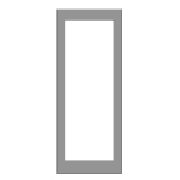
# Autodesk Inventor part: 50x40x3
Saved by Autodesk Inventor 2021 (Build 250183000, 183)
## iProperties
IsCustomPart: 1
Created: 2021-01-06
Part Number: 50x40x3
Material: Aluminum 6061
Document SubType Name: Modeling
Standard: Unnamed
Designer: lucky
Language: en-US
Size Designation: 50 x40 x3
Categories: <MemberInstance><Categories><Category DisplayName="Structural Shapes" InternalName="089c4875-fa83-4c05-b084-43b9cc11f5ed" Mnemonic="GRDR"><CategoryParameter DisplayName="Mass per Length Unit" InternalName="0bb95a10-148f-4027-a459-38d7b056702a" Mnemonic="shpmass"/><CategoryParameter DisplayName="Section Area" InternalName="1ff91680-64b0-4202-b9a3-7fd3f94bba3b" Mnemonic="secarea"/><CategoryParameter DisplayName="Radius of Gyration (x)" InternalName="25778675-03e9-40c1-b6a8-4a9ed693320d" Mnemonic="gyrradx"/><CategoryParameter DisplayName="Torsional Rigidity Modulus" InternalName="26c1ec35-5026-4c63-ad0a-751cf684a536" Mnemonic="torrigmod"/><CategoryParameter DisplayName="Distance of the Center of Gravity X-X" InternalName="26c9bdb8-9c79-4b4f-a92e-8e197583c9c4" Mnemonic="grcendistX"/><CategoryParameter DisplayName="Legacy Member ID" InternalName="340afe4f-75d7-48d3-ab7d-943f3c3da468" Mnemonic="LegacyMemberID"/><CategoryParameter DisplayName="Base Length" InternalName="42e34263-8f20-4d0e-ad48-bf1385b87c24" Mnemonic="shplen"/><CategoryParameter DisplayName="Moment of Inertia (y)" InternalName="4b9f58ea-bced-460e-81ea-3d29ca5a49e3" Mnemonic="inermomy"/><CategoryParameter DisplayName="Moment of Inertia (x)" InternalName="4cd780bc-73d7-43ac-917a-579e5cbd684d" Mnemonic="inermomx"/><CategoryParameter DisplayName="Custom Base Point" InternalName="4f1d1b73-316d-484b-a3df-9cbabb16eb77" Mnemonic="shpBasePoint"/><CategoryParameter DisplayName="Shape Height" InternalName="50274e7d-5ac0-4796-92cb-c59e54983c67" Mnemonic="shpheig"/><CategoryParameter DisplayName="Section Module (y)" InternalName="59eaa5e9-d227-48dc-b6c1-6920f96e0f95" Mnemonic="secmody"/><CategoryParameter DisplayName="Section Designation" InternalName="5a64d034-428d-49c8-ba32-7619764de20f" Mnemonic="shpdes"/><CategoryParameter DisplayName="Section Module (x)" InternalName="72cfad18-cf51-4ed4-aaa7-c6b224f8419f" Mnemonic="secmodx"/><CategoryParameter DisplayName="Torsional Section Modulus" InternalName="7c55a8dc-8844-49f9-a867-cc677b30ec9a" Mnemonic="torsecmod"/><CategoryParameter DisplayName="Shape Width" InternalName="7c717d54-a18f-4666-b4d4-573cce22c62c" Mnemonic="shpwdth"/><CategoryParameter DisplayName="Second Shape Thickness" InternalName="9251a8e1-85fd-4e47-af99-afdb762317d9" Mnemonic="shpthick2"/><CategoryParameter DisplayName="FG Authored" InternalName="9c666724-f362-4ea7-ac62-f6a007de5c69" Mnemonic="shpFGAuto"/><CategoryParameter DisplayName="Distance of the Center of Gravity Y-Y" InternalName="bcc4fb17-7af4-436a-8f8c-d0aa3b0248c5" Mnemonic="grcendistY"/><CategoryParameter DisplayName="Radius of Gyration (y)" InternalName="bfa18ebe-1636-4dbe-8d42-b263e0b73184" Mnemonic="gyrrady"/><CategoryParameter DisplayName="Shape Thickness" InternalName="d109cf76-8eb4-42fc-9800-4409734adc67" Mnemonic="shpthick"/><CategoryParameter DisplayName="Coefficient of Shear Displacement" InternalName="de4c90c6-aaa8-468f-a335-6737b311b5d3" Mnemonic="shdispc"/><Category DisplayName="Square/Rectangular Tubes" InternalName="afc8e2d8-05d6-4609-8807-f98a9b7d2ed0" Mnemonic="SQRSHP"><CategoryParameter DisplayName="Section Area" InternalName="2f7f79dd-983c-4263-802a-5b6a1495fdc5" Mnemonic="secarea"/><CategoryParameter DisplayName="Section Module (x)" InternalName="50d965a6-04bf-46b9-8ace-861858d348e6" Mnemonic="secmodx"/><CategoryParameter DisplayName="Section Module (y)" InternalName="5106aeac-54a2-4159-a9af-8933dd39dba2" Mnemonic="secmody"/><CategoryParameter DisplayName="Shape Thickness" InternalName="52712fc5-f4ee-4eda-b3f2-6fce82c26419" Mnemonic="shpthick"/><CategoryParameter DisplayName="Moment of Inertia (y)" InternalName="55ec8510-8276-4c45-8f10-594e0fee7eb3" Mnemonic="inermomy"/><CategoryParameter DisplayName="Radius of Gyration (x)" InternalName="56c89926-a299-4389-a862-ac94c9691272" Mnemonic="gyrradx"/><CategoryParameter DisplayName="Radius" InternalName="5d8d062c-e28e-41c1-98da-8e5fee36da1a" Mnemonic="shprad"/><CategoryParameter DisplayName="Moment of Inertia (x)" InternalName="8c4637b6-6b69-4878-9d5d-26a32185d655" Mnemonic="inermomx"/><CategoryParameter DisplayName="Shape Width" InternalName="8c8a1782-5e80-4d77-858b-304b1c0ad1fd" Mnemonic="shpwdth"/><CategoryParameter DisplayName="Radius of Gyration (y)" InternalName="fa48a7f5-f030-40f9-a60b-de8a845b7104" Mnemonic="gyrrady"/></Category></Category><Category DisplayName="DataType" InternalName="23b78d0f-2648-40c6-8793-ca6db495c9e8" Mnemonic="DATATYPE"><CategoryParameter DisplayName="DisplayName" InternalName="05415f3d-3907-474b-a020-eb9d644f4cf3" Mnemonic="DISPLAYNAME"/><CategoryParameter DisplayName="Standard" InternalName="0c0a119c-1e12-4c84-803f-101930972f5e" Mnemonic="STANDARD"/><CategoryParameter DisplayName="Description" InternalName="13903e3d-64b1-4950-80da-f627842ea37f" Mnemonic="DESCRIPTION"/><CategoryParameter DisplayName="Designation" InternalName="2675968c-4ce5-49e0-a4f5-552d29089031" Mnemonic="DESIGNATION"/><CategoryParameter DisplayName="Default Row" InternalName="2af9ec52-faaa-4026-b378-f9fa4afca842" Mnemonic="DEFAULTROW"/><CategoryParameter DisplayName="Folder Name" InternalName="3f06958e-8713-4116-9be7-ed6184ecc97b" Mnemonic="FOLDERNAME"/><CategoryParameter DisplayName="Revision Guid" InternalName="45a75005-10b1-4dfc-8d6d-dfe629f0b93c" Mnemonic="REVISIONGUID"/><CategoryParameter DisplayName="FileName" InternalName="8b46a4cc-9585-4fed-90c3-899f57e09a73" Mnemonic="FILENAME"/><CategoryParameter DisplayName="StdsOrg" InternalName="8f5914e1-4693-403f-8ab5-d37768198c9d" Mnemonic="STDSORG"/><CategoryParameter DisplayName="Family Version" InternalName="914462f6-6e19-4b14-ba84-155b9680b1d0" Mnemonic="FAMILYREVISION"/><CategoryParameter DisplayName="Standard Revision" InternalName="91d5a463-65c2-4fde-b823-3b7fea5e8e17" Mnemonic="STANDARDREVISION"/><CategoryParameter DisplayName="Member Revision" InternalName="a65d44b9-392f-4f4f-857b-e4b3d54996fe" Mnemonic="MEMBERREVISION"/><CategoryParameter DisplayName="ClipFormat" InternalName="bc51e27b-3422-4e78-93ef-cec197ddf230" Mnemonic="CLIPFORMAT"/><CategoryParameter DisplayName="Manufacturer" InternalName="cd6c7a72-a28a-4e50-99a9-2c7f4e13e5ad" Mnemonic="MANUFACTURER"/><CategoryParameter DisplayName="InternalName" InternalName="cf1d0246-76d9-4b4a-8305-fa0409afb5c1" Mnemonic="INTERNALNAME"/><CategoryParameter DisplayName="IsMetric" InternalName="e2385c5b-1ea4-4823-96a8-8de651266ec3" Mnemonic="ISMETRIC"/><Category DisplayName="Part" InternalName="c0e0b642-3bcb-4cc8-9e80-f96d35c4afa4" Mnemonic="PART"><CategoryParameter DisplayName="Part Number" InternalName="016b6077-bfbe-49bd-92c9-d8d59c39c941" Mnemonic="PARTNUMBER"/><CategoryParameter DisplayName="Stock Number" InternalName="4dba7c1c-e26c-444e-836c-b08b433409a8" Mnemonic="STOCKNUMBER"/><CategoryParameter DisplayName="Material Key" InternalName="5c9a8adb-dd2b-4535-b97f-0a94a95fe41f" Mnemonic="MATERIALKEY"/><CategoryParameter DisplayName="Material" InternalName="818a152a-d3c3-49ca-80ee-df7d91421b8e" Mnemonic="MATERIAL"/></Category></Category></Categories><FamilyTemplate Id="ALUMINIUM SECTION"><FamilyTemplateParameters><FamilyTemplateParameter ObjectType="kUserParameterObject" ValueType="xs:double" Id="1" ObjectReferenceKey="G_L"/><FamilyTemplateParameter ObjectType="kUserParameterObject" ValueType="xs:double" Id="2" ObjectReferenceKey="G_OFFSET_END"/><FamilyTemplateParameter ObjectType="kUserParameterObject" ValueType="xs:double" Id="3" ObjectReferenceKey="G_OFFSET_START"/><FamilyTemplateParameter ObjectType="kUserParameterObject" ValueType="xs:double" Id="4" ObjectReferenceKey="Height"/><FamilyTemplateParameter ObjectType="kModelParameterObject" ValueType="xs:double" Id="5" ObjectReferenceKey="Length"/><FamilyTemplateParameter ObjectType="kUserParameterObject" ValueType="xs:double" Id="7" ObjectReferenceKey="Thickness"/><FamilyTemplateParameter ObjectType="kUserParameterObject" ValueType="xs:double" Id="8" ObjectReferenceKey="Width"/><FamilyTemplateParameter ObjectType="kPartComponentDefinitionObject" ValueType="xs:string" Id="10" SubObjectId="Material"/><FamilyTemplateParameter ObjectType="kPropertyObject" ValueType="xs:string" Id="22" ObjectReferenceKey="{32853F0F-3444-11d1-9E93-0060B03C1CA6}" SubObjectId="5"/><FamilyTemplateParameter ObjectType="kPropertyObject" ValueType="xs:string" Id="23" ObjectReferenceKey="{32853F0F-3444-11d1-9E93-0060B03C1CA6}" SubObjectId="52"/></FamilyTemplateParameters></FamilyTemplate><CategoryParameterMap><ParamToTemplateMap><ParamToTemplate CategoryParameter="//CategoryParameter[@InternalName='cf1d0246-76d9-4b4a-8305-fa0409afb5c1']" ConstantValue="15910203-61a6-416b-84d3-bf7a968be789"/><ParamToTemplate CategoryParameter="//CategoryParameter[@InternalName='45a75005-10b1-4dfc-8d6d-dfe629f0b93c']" ConstantValue="f0420af0-eaa1-4c46-be67-1e58856612a2"/><ParamToTemplate CategoryParameter="//CategoryParameter[@InternalName='3f06958e-8713-4116-9be7-ed6184ecc97b']" ConstantValue="ALUMINIUM SECTION"/><ParamToTemplate CategoryParameter="//CategoryParameter[@InternalName='8f5914e1-4693-403f-8ab5-d37768198c9d']" TemplateParameter="15"/><ParamToTemplate CategoryParameter="//CategoryParameter[@InternalName='0c0a119c-1e12-4c84-803f-101930972f5e']" TemplateParameter="16"/><ParamToTemplate CategoryParameter="//CategoryParameter[@InternalName='91d5a463-65c2-4fde-b823-3b7fea5e8e17']" TemplateParameter="17"/><ParamToTemplate CategoryParameter="//CategoryParameter[@InternalName='cd6c7a72-a28a-4e50-99a9-2c7f4e13e5ad']" TemplateParameter="18"/><ParamToTemplate CategoryParameter="//CategoryParameter[@InternalName='13903e3d-64b1-4950-80da-f627842ea37f']" TemplateParameter="19"/><ParamToTemplate CategoryParameter="//CategoryParameter[@InternalName='05415f3d-3907-474b-a020-eb9d644f4cf3']" ConstantValue="ALUMINIUM SECTION"/><ParamToTemplate CategoryParameter="//CategoryParameter[@InternalName='914462f6-6e19-4b14-ba84-155b9680b1d0']" ConstantValue="11"/><ParamToTemplate CategoryParameter="//CategoryParameter[@InternalName='bc51e27b-3422-4e78-93ef-cec197ddf230']" ConstantValue="CF_INVENTOR.STDPARTS"/><ParamToTemplate CategoryParameter="//CategoryParameter[@InternalName='e2385c5b-1ea4-4823-96a8-8de651266ec3']" ConstantValue="true"/><ParamToTemplate CategoryParameter="//CategoryParameter[@InternalName='2af9ec52-faaa-4026-b378-f9fa4afca842']" ConstantValue="1"/><ParamToTemplate CategoryParameter="//CategoryParameter[@InternalName='9c666724-f362-4ea7-ac62-f6a007de5c69']" ConstantValue="1"/><ParamToTemplate CategoryParameter="//CategoryParameter[@InternalName='8b46a4cc-9585-4fed-90c3-899f57e09a73']" ConstantValue="ALUMINIUM RHS 25x50x3"/><ParamToTemplate CategoryParameter="//CategoryParameter[@InternalName='a65d44b9-392f-4f4f-857b-e4b3d54996fe']" ConstantValue="1256fa95-0645-45ac-8834-58378d85df9d"/><ParamToTemplate CategoryParameter="//CategoryParameter[@InternalName='a65d44b9-392f-4f4f-857b-e4b3d54996fe']" ConstantValue="1256fa95-0645-45ac-8834-58378d85df9d"/><ParamToTemplate CategoryParameter="//CategoryParameter[@InternalName='2675968c-4ce5-49e0-a4f5-552d29089031']" TemplateParameter="23"/><ParamToTemplate CategoryParameter="//CategoryParameter[@InternalName='50274e7d-5ac0-4796-92cb-c59e54983c67']" TemplateParameter="4"/><ParamToTemplate CategoryParameter="//CategoryParameter[@InternalName='42e34263-8f20-4d0e-ad48-bf1385b87c24']" TemplateParameter="5"/><ParamToTemplate CategoryParameter="//CategoryParameter[@InternalName='818a152a-d3c3-49ca-80ee-df7d91421b8e']" TemplateParameter="10"/><ParamToTemplate CategoryParameter="//CategoryParameter[@InternalName='016b6077-bfbe-49bd-92c9-d8d59c39c941']" TemplateParameter="22"/><ParamToTemplate CategoryParameter="//CategoryParameter[@InternalName='52712fc5-f4ee-4eda-b3f2-6fce82c26419']" TemplateParameter="7"/><ParamToTemplate CategoryParameter="//CategoryParameter[@InternalName='7c717d54-a18f-4666-b4d4-573cce22c62c']" TemplateParameter="8"/></ParamToTemplateMap></CategoryParameterMap></MemberInstance>
Density: 2.7 g/cm^3
Appearance: Aluminum - Flat
Mass: 782.883 g
Surface Area: 2002.24 cm^2
Volume: 289.957 cm^3
_CCFamilyDisplayName: ALUMINIUM SECTION -
_FrameMemberDoc: Frame Member File
_Version: 25.0.0
_GetPNFromCC: 1
G_W: 40.000 mm
G_H: 50.000 mm
+E11D9175-CA95-43D0-AAAB-BDCB84E0D158+CUTDETAIL3: Cut Angle 90.00 deg
G_L: 750.000 mm
+0628A439-B4A6-4B13-AF6A-39B941D8A988+CUTDETAIL4: Cut Angle 90.00 deg
Author: lucky
Autodesk Inventor part; units mm, degrees
ref_plane "Start Plane" through (0, 0, 25) normal (0, 0, 1) x (1, 0, 0)
ref_plane "End Plane" through (0, 0, 775) normal (0, 0, 1) x (1, 0, 0)
sketch "Sketch" plane through (0, 0, 0) normal (0, 0, 1) x (1, 0, 0)
  line L0 (-20, -25) -> (20, -25)
  line L1 (20, -25) -> (20, 25)
  line L2 (20, 25) -> (-20, 25)
  line L3 (-20, 25) -> (-20, -25)
  line L4 (-20, -25) -> (20, 25) construction
  line L5 (20, -25) -> (-20, 25) construction
  line L6 (-17, 22) -> (17, 22)
  line L7 (17, 22) -> (17, -22)
  line L8 (17, -22) -> (-17, -22)
  line L9 (-17, -22) -> (-17, 22)
  point P0 (0, 0)
  dimension "Width" = 40
  dimension "Height" = 50
  dimension "Thickness" = 3
  constraints: 20 end point, 4 parallel, 2 midpoint, 2 perpendicular, 1 horizontal, 3 other
  measures "Width" distance between parallel lines of L1 L3
  measures "Height" distance of L0.end L1.end
  measures "Thickness" distance between parallel lines of L2 L6
extrude "Body" add sketch "Sketch" along normal up to surface (750 mm away) from surface at 25
sketch "Sketch2" plane through (0, 0, 0) normal (0, 0, 1) x (1, 0, 0)
  line L0 (0, 0) -> (10, 0)
ref_plane "Work Plane3" through (0, 0, 0) normal (0, -1, 0) x (1, 0, 0)
sketch "Sketch3" plane through (0, 0, 0) normal (0, -1, 0) x (1, 0, 0)
  line L0 (-28, 25) -> (28, 25)
  line L1 (-28, 775) -> (28, 775)
  dimension "d10" = 750
  measures "d10" distance between parallel lines of L0 L1
ref_plane "Work Plane5" through (628, -25, 25) normal (0, 0, -1) x (-1, 0, 0)
split "Split2" plane through (628, -25, 25) removes the side toward (0, 0, -1)
ref_plane "Work Plane6" through (-72, -25, 775) normal (0, 0, 1) x (1, 0, 0)
split "Split3" plane through (-72, -25, 775) removes the side toward (0, 0, 1)
sketch "Sketch4" plane through (-20, -25, 775) normal (-1, 0, 0) x (0, 0, 1)
  line L0 (-750, 50) -> (0, 50) projected
  line L1 (-750, 0) -> (0, 0) projected
  line L2 (-660.75, 18.2875) -> (-89.25, 18.2875)
  line L3 (-750, 3) -> (-750, 47) construction
  line L4 (-750, 25) -> (0, 25) construction
  line L5 (0, 3) -> (0, 47) construction
  line L6 (-750, 0) -> (-750, 50) projected
  line L7 (0, 0) -> (0, 50) projected
  point P0 (-775, 25)
  point P1 (-375, 18.2875)
  point P2 (-375, 0)
  dimension "d11" = 571.5
  dimension "d44" = 18.2875
  constraints: 4 end point, 4 midpoint, 1 coincident, 1 horizontal, 1 vertical alignment
  measures "d11" distance of L2.start L2.end
  measures "d44" distance between parallel lines of L1 L2
hole "Hole1" at (-20, -6.7125, 114.25) direction (1, 0, 0) diameter 28.575 end through all
pattern_linear "Rectangular Pattern1" count 3 spacing 285.75 along (0, 0, 1) of "Hole1"
sketch "Sketch5" plane through (-20, -25, 775) normal (-1, 0, 0) x (0, 0, 1)
  line L0 (0, 0) -> (0, 50) projected
  line L1 (-750, 50) -> (0, 50) projected
  line L2 (-750, 0) -> (-750, 50) projected
  line L3 (-750, 0) -> (0, 0) projected
  line L4 (-775, 25) -> (25, 25)
  point P0 (-375, 17)
  point P1 (-375, 19.9091)
  point P2 (-375, 25)
  point P3 (-375, 25)
  dimension "d35" = 8
  constraints: 3 vertical alignment, 2 end point, 1 horizontal, 1 midpoint, 2 other
  measures "d35" distance from line of L4 point (-375, 17)
hole "Hole2" [suppressed]
sketch "Sketch7" plane through (-20, -25, 775) normal (-1, 0, 0) x (0, 0, 1)
  line L0 (-666.5, 21) -> (-83.5, 21) construction
  line L1 (-766.8103, 25) -> (25, 25) construction
  point P0 (-375, 21)
  point P1 (-375, 25)
  dimension "d36" = 583
  dimension "d40" = 4
  constraints: 4 end point, 2 horizontal, 1 midpoint, 1 vertical alignment, 2 other
  measures "d36" distance of L0.end L0.start
  measures "d40" distance between parallel lines of L1 L0
pattern_linear "Rectangular Pattern2" count 4 spacing 190.5 along (0, 0, 1) of "Hole1"
sketch "Sketch9" plane through (20, -25, 775) normal (1, 0, 0) x (0, 0, -1)
  line L0 (0, 50) -> (750, 50) projected
  line L1 (750, 0) -> (750, 50) projected
  line L2 (0, 50) -> (750, 50) projected
  line L3 (0, 0) -> (0, 50) projected
  line L4 (0, 0) -> (750, 0) projected
  circle A0 centre (660.8, 18.2875) radius 12.7 projected
  circle A1 centre (279.75, 18.2875) radius 14.2875 projected
  circle A2 centre (470.25, 18.2875) radius 14.2875 projected
  circle A3 centre (660.75, 18.2875) radius 14.2875 projected
  circle A4 centre (375, 18.2875) radius 14.2875 projected
  circle A5 centre (89.25, 18.2875) radius 14.2875 projected
  point P0 (775, 25)
  point P1 (565.5644, 19.942)
  dimension "d57" = 95.25
  dimension "d58" = 30.058
  measures "d57" distance of point (565.564, 19.942) A0.centre
  measures "d58" distance from line of L0 point (565.564, 19.942)
hole "Hole4" at (20, -5.058, 209.4356) direction (-1, 0, 0) diameter 28.575 depth 10
sketch "Sketch12" plane through (17, -25, 775) normal (-1, 0, 0) x (0, 0, 1)
  point P0 (-775, 25)
sketch "Sketch13" plane through (-20, -25, 775) normal (0, -1, 0) x (1, 0, 0)
  line L0 (0, -750) -> (0, 0) projected
  line L1 (3, -750) -> (3, 0) projected
  line L2 (37, -750) -> (37, 0) projected
  line L3 (-55, -750) -> (645, -750) projected
  line L4 (-55, 0) -> (645, 0) projected
  line L5 (37, -750) -> (37, 0) projected
  line L6 (3, -710.75) -> (37, -710.75)
  line L7 (37, -710.75) -> (37, -39.25)
  line L8 (37, -39.25) -> (3, -39.25)
  line L9 (3, -39.25) -> (3, -710.75)
  point P0 (20, -775)
  point P1 (37, -375)
  point P2 (37, -375)
  point P3 (37, -39.25)
  point P4 (3, -39.25)
  point P5 (37, -710.75)
  dimension "d73" = 671.5
  constraints: 8 end point, 2 midpoint, 2 parallel, 2 point on line, 1 coincident, 1 horizontal, 1 perpendicular
  measures "d73" distance between parallel lines of L8 L6
extrude "Extrusion4" cut sketch "Sketch13" against normal blind 10 contours L1 L8 L2 L6
sketch "Sketch14" plane through (20, -25, 775) normal (1, 0, 0) x (0, 0, -1)
  circle A0 centre (375, 18.2875) radius 14.2875 projected
  point P0 (775, 25)
equation "\"d22\" = Wheel_Seperation"
equation "\"d35\" = Wheel_HeightOffset + Wheel_CentreDrop"
equation "\"d36\" = 3 * Wheel_Seperation2"
equation "\"d40\" = Wheel_HeightOffset2"
equation "\"d43\" = Wheel_MaxSeperation2"
equation "\"d57\" = MotorholeCC"
equation "\"d58\" = OutputshaftTopOffset"
equation "\"G_OFFSET_START\" = -25"
equation "\"G_OFFSET_END\" = -25"
equation "\"d5\" = -G_OFFSET_START"
equation "\"d6\" = Length + G_OFFSET_END"
equation "\"G_L\" = 750"
equation "\"Chassi_CentreDrop\" = 4"
equation "\"WheelBay_Depth\" = 55"
equation "\"Wheel_Diametre\" = 152.4"
equation "\"Wheel_Seperation\" = 285.75"
equation "\"Wheel_HeightOffset\" = 4"
equation "\"Wheel_Clearance\" = 13.05"
equation "\"Chassi_GroundClearance\" = 10.116"
equation "\"Wheel_CentreDrop\" = 4"
equation "\"Wheel_Seperation2\" = 194.33333"
equation "\"Wheel_Diametre2\" = 101.6"
equation "\"Wheel_HeightOffset2\" = 4"
equation "\"Wheel_Clearance2\" = 32.7"
equation "\"Chain_Pitch\" = 9.525"
equation "\"Wheel_MaxSeperation\" = 285.75"
equation "\"Wheel_CCSpan\" = 571.5"
equation "\"Wheel_CCSpan2\" = 471.5"
equation "\"Wheel_MaxSeperation2\" = 190.5"
equation "\"MotorholeCC\" = 95.25"
equation "\"MotorholeHorizontal\" = 95.01318"
equation "\"OutputshaftTopOffset\" = 30.058"
equation "\"Heightfromcenter\" = 6.7125"
equation "\"Chassi_SideRivetSpacing\" = 37.5"
equation "\"Sprocket_Thickness\" = 10.668"
equation "\"BumperMountingBarOffset\" = 177.8"
equation "\"Length\" = 800"
body "Solid1"
